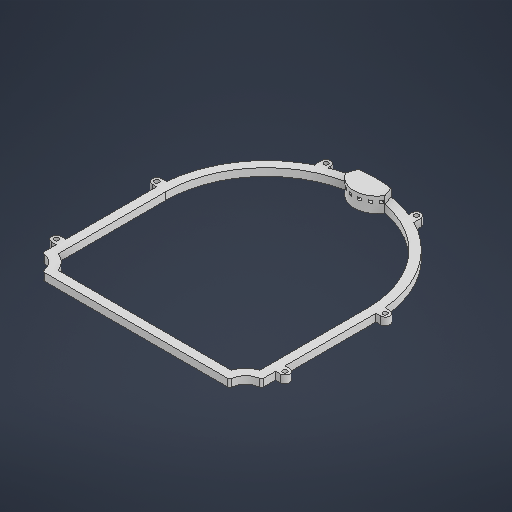
# Autodesk Inventor part: acrylic_clamp
Saved by Autodesk Inventor 2026.2 (Build 302298000, 298)
## iProperties
Created: 2026-04-07
Part Number: acrylic_clamp
Material: Generic
Document SubType Name: Modeling
Designer: Tathagata Sikdar
Density: 1 g/cm^3
Appearance: Default
Author: Tathagata Sikdar
Autodesk Inventor part; units mm, degrees
ref_plane "YZ Plane" through (0, 0, 0) normal (1, 0, 0) x (0, 1, 0)
ref_plane "Work Plane1" through (-76.1962, 17.6834, 72.2477) normal (0, 1, 0) x (-1, 0, 0)
sketch "Sketch1" plane through (-76.1962, 17.6834, 72.2477) normal (0, 1, 0) x (-1, 0, 0)
  arc A0 (-12.9956, -95.0875) -> (-10.7767, -93.6645) centre (-12.6982, -93.1097) ccw projected
  arc A1 (10.7767, -93.6645) -> (-10.7767, -93.6645) centre (0, -96.776) ccw projected
  arc A2 (10.7767, -93.6645) -> (12.9956, -95.0875) centre (12.6982, -93.1097) ccw projected
  arc A3 (12.9956, -95.0875) -> (32.2927, -89.8741) centre (0, -8.6647) ccw projected
  line L0 (32.2927, -89.8741) -> (32.2927, -92.3799) projected
  arc A4 (32.2927, -92.3799) -> (39.7927, -92.3799) centre (36.0427, -92.3799) ccw projected
  line L1 (39.7927, -92.3799) -> (39.7927, -86.4742) projected
  arc A5 (39.7927, -86.4742) -> (87.075, -16.1299) centre (0, -8.6647) ccw projected
  line L2 (87.075, -16.1299) -> (91.0687, -16.1299) projected
  arc A6 (91.0687, -16.1299) -> (91.0687, -8.6299) centre (91.0687, -12.3799) ccw projected
  line L3 (91.0687, -8.6299) -> (87.3944, -8.6299) projected
  line L4 (87.3944, -8.6299) -> (87.3944, 63.8701) projected
  line L5 (87.3944, 63.8701) -> (91.1444, 63.8701) projected
  arc A7 (91.1444, 63.8701) -> (91.1444, 71.3701) centre (91.1444, 67.6201) ccw projected
  line L6 (91.1444, 71.3701) -> (87.3944, 71.3701) projected
  line L7 (87.3944, 71.3701) -> (87.3944, 80.7566) projected
  arc A8 (87.3944, 80.7566) -> (85.666, 82.738) centre (85.3944, 80.7566) ccw projected
  arc A9 (74.7844, 93.6197) -> (85.666, 82.738) centre (87.3944, 95.3481) ccw projected
  arc A10 (74.7844, 93.6197) -> (72.8029, 95.3481) centre (72.8029, 93.3481) ccw projected
  line L8 (72.8029, 95.3481) -> (-72.8029, 95.3481) projected
  arc A11 (-72.8029, 95.3481) -> (-74.7844, 93.6197) centre (-72.8029, 93.3481) ccw projected
  arc A12 (-85.666, 82.738) -> (-74.7844, 93.6197) centre (-87.3944, 95.3481) ccw projected
  arc A13 (-85.666, 82.738) -> (-87.3944, 80.7566) centre (-85.3944, 80.7566) ccw projected
  line L9 (-87.3944, 80.7566) -> (-87.3944, 71.3701) projected
  line L10 (-87.3944, 71.3701) -> (-91.1444, 71.3701) projected
  arc A14 (-91.1444, 71.3701) -> (-91.1444, 63.8701) centre (-91.1444, 67.6201) ccw projected
  line L11 (-91.1444, 63.8701) -> (-87.3944, 63.8701) projected
  line L12 (-87.3944, 63.8701) -> (-87.3944, -8.6299) projected
  line L13 (-87.3944, -8.6299) -> (-91.1444, -8.6299) projected
  arc A15 (-91.1444, -8.6299) -> (-91.1444, -16.1299) centre (-91.1444, -12.3799) ccw projected
  line L14 (-91.1444, -16.1299) -> (-87.075, -16.1299) projected
  arc A16 (-87.075, -16.1299) -> (-39.7927, -86.4742) centre (0, -8.6647) ccw projected
  line L15 (-39.7927, -86.4742) -> (-39.7927, -92.3799) projected
  arc A17 (-39.7927, -92.3799) -> (-32.2927, -92.3799) centre (-36.0427, -92.3799) ccw projected
  line L16 (-32.2927, -92.3799) -> (-32.2927, -89.8741) projected
  arc A18 (-32.2927, -89.8741) -> (-12.9956, -95.0875) centre (0, -8.6647) ccw projected
  circle A19 centre (-36.0427, -92.3799) radius 1.85 projected
  circle A20 centre (91.1444, 67.6201) radius 1.85 projected
  circle A21 centre (36.0427, -92.3799) radius 1.85 projected
  circle A22 centre (-91.1444, 67.6201) radius 1.85 projected
  circle A23 centre (-91.1444, -12.3799) radius 1.85 projected
  circle A24 centre (91.0687, -12.3799) radius 1.85 projected
  arc A25 (85.9744, 79.5665) -> (84.398, 81.5211) centre (83.9744, 79.5665) ccw projected
  line L17 (85.9744, 79.5665) -> (85.9744, -8.6647) projected
  arc A26 (13.9862, -93.4939) -> (85.9744, -8.6647) centre (0, -8.6647) ccw projected
  arc A27 (11.7942, -92.2386) -> (13.9862, -93.4939) centre (13.6608, -91.5205) ccw projected
  arc A28 (11.7942, -92.2386) -> (-11.7942, -92.2386) centre (0, -96.776) ccw projected
  arc A29 (-13.9862, -93.4939) -> (-11.7942, -92.2386) centre (-13.6608, -91.5205) ccw projected
  arc A30 (-85.9744, -8.6647) -> (-13.9862, -93.4939) centre (0, -8.6647) ccw projected
  line L18 (-85.9744, -8.6647) -> (-85.9744, 79.5665) projected
  arc A31 (-84.398, 81.5211) -> (-85.9744, 79.5665) centre (-83.9744, 79.5665) ccw projected
  arc A32 (-84.398, 81.5211) -> (-73.5675, 92.3516) centre (-87.3944, 95.3481) ccw projected
  arc A33 (-71.6128, 93.9281) -> (-73.5675, 92.3516) centre (-71.6128, 91.9281) ccw projected
  line L19 (-71.6128, 93.9281) -> (71.6128, 93.9281) projected
  arc A34 (73.5675, 92.3516) -> (71.6128, 93.9281) centre (71.6128, 91.9281) ccw projected
  arc A35 (73.5675, 92.3516) -> (84.398, 81.5211) centre (87.3944, 95.3481) ccw projected
  arc A36 (14.2722, -87.9193) -> (-14.2722, -87.9193) centre (0, -96.776) ccw projected
  arc A37 (14.2722, -87.9193) -> (16.3718, -88.8243) centre (15.9716, -86.8648) ccw projected
  arc A38 (16.3718, -88.8243) -> (81.8144, -8.6647) centre (0, -8.6647) ccw projected
  line L20 (81.8144, -8.6647) -> (81.8144, 76.5078) projected
  arc A39 (81.8144, 76.5078) -> (80.5609, 78.3633) centre (79.8144, 76.5078) ccw projected
  arc A40 (70.4096, 88.5146) -> (80.5609, 78.3633) centre (87.3944, 95.3481) ccw projected
  arc A41 (70.4096, 88.5146) -> (68.5542, 89.7681) centre (68.5542, 87.7681) ccw projected
  line L21 (68.5542, 89.7681) -> (-68.5542, 89.7681) projected
  arc A42 (-68.5542, 89.7681) -> (-70.4096, 88.5146) centre (-68.5542, 87.7681) ccw projected
  arc A43 (-80.5609, 78.3633) -> (-70.4096, 88.5146) centre (-87.3944, 95.3481) ccw projected
  arc A44 (-80.5609, 78.3633) -> (-81.8144, 76.5078) centre (-79.8144, 76.5078) ccw projected
  line L22 (-81.8144, 76.5078) -> (-81.8144, -8.6647) projected
  arc A45 (-81.8144, -8.6647) -> (-16.3718, -88.8243) centre (0, -8.6647) ccw projected
  arc A46 (-16.3718, -88.8243) -> (-14.2722, -87.9193) centre (-15.9716, -86.8648) ccw projected
  arc A47 (15.6866, -87.5139) -> (80.3944, -8.6647) centre (0, -8.6647) ccw projected
  arc A48 (15.6866, -87.5139) -> (-15.6866, -87.5139) centre (0, -96.776) ccw projected
  arc A49 (-80.3944, -8.6647) -> (-15.6866, -87.5139) centre (0, -8.6647) ccw projected
  line L23 (-80.3944, -8.6647) -> (-80.3944, 76.9038) projected
  arc A50 (-80.3944, 76.9038) -> (-68.9502, 88.3481) centre (-87.3944, 95.3481) ccw projected
  line L24 (-68.9502, 88.3481) -> (68.9502, 88.3481) projected
  arc A51 (68.9502, 88.3481) -> (80.3944, 76.9038) centre (87.3944, 95.3481) ccw projected
  line L25 (80.3944, 76.9038) -> (80.3944, -8.6647) projected
  point P0 (-76.1962, -72.2477)
extrude "Extrusion1" add sketch "Sketch1" along normal blind 6
sketch "Sketch2" plane through (-76.1962, 23.6834, 72.2477) normal (0, 1, 0) x (1, 0, 0)
  line L0 (87.3944, -80.7566) -> (87.3944, -71.3701) projected
  line L1 (87.3944, -71.3701) -> (91.1444, -71.3701) projected
  arc A0 (91.1444, -71.3701) -> (91.1444, -63.8701) centre (91.1444, -67.6201) ccw projected
  line L2 (91.1444, -63.8701) -> (87.3944, -63.8701) projected
  line L3 (87.3944, -63.8701) -> (87.3944, 8.6299) projected
  line L4 (87.3944, 8.6299) -> (91.1444, 8.6299) projected
  arc A1 (91.1444, 8.6299) -> (91.1444, 16.1299) centre (91.1444, 12.3799) ccw projected
  line L5 (91.1444, 16.1299) -> (87.075, 16.1299) projected
  arc A2 (87.075, 16.1299) -> (39.7927, 86.4742) centre (0, 8.6647) ccw projected
  line L6 (39.7927, 86.4742) -> (39.7927, 92.3799) projected
  arc A3 (39.7927, 92.3799) -> (32.2927, 92.3799) centre (36.0427, 92.3799) ccw projected
  line L7 (32.2927, 92.3799) -> (32.2927, 89.8741) projected
  arc A4 (32.2927, 89.8741) -> (12.9956, 95.0875) centre (0, 8.6647) ccw projected
  arc A5 (12.9956, 95.0875) -> (10.7767, 93.6645) centre (12.6982, 93.1097) ccw projected
  arc A6 (-10.7767, 93.6645) -> (10.7767, 93.6645) centre (0, 96.776) ccw projected
  arc A7 (-10.7767, 93.6645) -> (-12.9956, 95.0875) centre (-12.6982, 93.1097) ccw projected
  arc A8 (-12.9956, 95.0875) -> (-32.2927, 89.8741) centre (0, 8.6647) ccw projected
  line L8 (-32.2927, 89.8741) -> (-32.2927, 92.3799) projected
  arc A9 (-32.2927, 92.3799) -> (-39.7927, 92.3799) centre (-36.0427, 92.3799) ccw projected
  line L9 (-39.7927, 92.3799) -> (-39.7927, 86.4742) projected
  arc A10 (-39.7927, 86.4742) -> (-87.075, 16.1299) centre (0, 8.6647) ccw projected
  line L10 (-87.075, 16.1299) -> (-91.0687, 16.1299) projected
  arc A11 (-91.0687, 16.1299) -> (-91.0687, 8.6299) centre (-91.0687, 12.3799) ccw projected
  line L11 (-91.0687, 8.6299) -> (-87.3944, 8.6299) projected
  line L12 (-87.3944, 8.6299) -> (-87.3944, -63.8701) projected
  line L13 (-87.3944, -63.8701) -> (-91.1444, -63.8701) projected
  arc A12 (-91.1444, -63.8701) -> (-91.1444, -71.3701) centre (-91.1444, -67.6201) ccw projected
  line L14 (-91.1444, -71.3701) -> (-87.3944, -71.3701) projected
  line L15 (-87.3944, -71.3701) -> (-87.3944, -80.7566) projected
  arc A13 (-87.3944, -80.7566) -> (-85.666, -82.738) centre (-85.3944, -80.7566) ccw projected
  arc A14 (-74.7844, -93.6197) -> (-85.666, -82.738) centre (-87.3944, -95.3481) ccw projected
  arc A15 (-74.7844, -93.6197) -> (-72.8029, -95.3481) centre (-72.8029, -93.3481) ccw projected
  line L16 (-72.8029, -95.3481) -> (72.8029, -95.3481) projected
  arc A16 (72.8029, -95.3481) -> (74.7844, -93.6197) centre (72.8029, -93.3481) ccw projected
  arc A17 (85.666, -82.738) -> (74.7844, -93.6197) centre (87.3944, -95.3481) ccw projected
  arc A18 (85.666, -82.738) -> (87.3944, -80.7566) centre (85.3944, -80.7566) ccw projected
  arc A19 (-11.7942, 92.2386) -> (11.7942, 92.2386) centre (0, 96.776) ccw projected
  arc A20 (13.9862, 93.4939) -> (11.7942, 92.2386) centre (13.6608, 91.5205) ccw projected
  arc A21 (85.9744, 8.6647) -> (13.9862, 93.4939) centre (0, 8.6647) ccw projected
  line L17 (85.9744, 8.6647) -> (85.9744, -79.5665) projected
  arc A22 (84.398, -81.5211) -> (85.9744, -79.5665) centre (83.9744, -79.5665) ccw projected
  arc A23 (84.398, -81.5211) -> (73.5675, -92.3516) centre (87.3944, -95.3481) ccw projected
  arc A24 (71.6128, -93.9281) -> (73.5675, -92.3516) centre (71.6128, -91.9281) ccw projected
  line L18 (71.6128, -93.9281) -> (-71.6128, -93.9281) projected
  arc A25 (-73.5675, -92.3516) -> (-71.6128, -93.9281) centre (-71.6128, -91.9281) ccw projected
  arc A26 (-73.5675, -92.3516) -> (-84.398, -81.5211) centre (-87.3944, -95.3481) ccw projected
  arc A27 (-85.9744, -79.5665) -> (-84.398, -81.5211) centre (-83.9744, -79.5665) ccw projected
  line L19 (-85.9744, -79.5665) -> (-85.9744, 8.6647) projected
  arc A28 (-13.9862, 93.4939) -> (-85.9744, 8.6647) centre (0, 8.6647) ccw projected
  arc A29 (-11.7942, 92.2386) -> (-13.9862, 93.4939) centre (-13.6608, 91.5205) ccw projected
  circle A30 centre (-91.0687, 12.3799) radius 1.85 projected
  circle A31 centre (91.1444, 12.3799) radius 1.85 projected
  circle A32 centre (91.1444, -67.6201) radius 1.85 projected
  circle A33 centre (-36.0427, 92.3799) radius 1.85 projected
  circle A34 centre (-91.1444, -67.6201) radius 1.85 projected
  circle A35 centre (36.0427, 92.3799) radius 1.85 projected
  line L20 (-81.8144, 8.6647) -> (-81.8144, -76.5078) projected
  arc A36 (-81.8144, -76.5078) -> (-80.5609, -78.3633) centre (-79.8144, -76.5078) ccw projected
  arc A37 (-70.4096, -88.5146) -> (-80.5609, -78.3633) centre (-87.3944, -95.3481) ccw projected
  arc A38 (-70.4096, -88.5146) -> (-68.5542, -89.7681) centre (-68.5542, -87.7681) ccw projected
  line L21 (-68.5542, -89.7681) -> (68.5542, -89.7681) projected
  arc A39 (68.5542, -89.7681) -> (70.4096, -88.5146) centre (68.5542, -87.7681) ccw projected
  arc A40 (80.5609, -78.3633) -> (70.4096, -88.5146) centre (87.3944, -95.3481) ccw projected
  arc A41 (80.5609, -78.3633) -> (81.8144, -76.5078) centre (79.8144, -76.5078) ccw projected
  line L22 (81.8144, -76.5078) -> (81.8144, 8.6647) projected
  arc A42 (81.8144, 8.6647) -> (16.3718, 88.8243) centre (0, 8.6647) ccw projected
  arc A43 (16.3718, 88.8243) -> (14.2722, 87.9193) centre (15.9716, 86.8648) ccw projected
  arc A44 (-14.2722, 87.9193) -> (14.2722, 87.9193) centre (0, 96.776) ccw projected
  arc A45 (-14.2722, 87.9193) -> (-16.3718, 88.8243) centre (-15.9716, 86.8648) ccw projected
  arc A46 (-16.3718, 88.8243) -> (-81.8144, 8.6647) centre (0, 8.6647) ccw projected
  line L23 (80.3944, 8.6647) -> (80.3944, -76.9038) projected
  arc A47 (80.3944, -76.9038) -> (68.9502, -88.3481) centre (87.3944, -95.3481) ccw projected
  line L24 (68.9502, -88.3481) -> (-68.9502, -88.3481) projected
  arc A48 (-68.9502, -88.3481) -> (-80.3944, -76.9038) centre (-87.3944, -95.3481) ccw projected
  line L25 (-80.3944, -76.9038) -> (-80.3944, 8.6647) projected
  arc A49 (-15.6866, 87.5139) -> (-80.3944, 8.6647) centre (0, 8.6647) ccw projected
  arc A50 (-15.6866, 87.5139) -> (15.6866, 87.5139) centre (0, 96.776) ccw projected
  arc A51 (80.3944, 8.6647) -> (15.6866, 87.5139) centre (0, 8.6647) ccw projected
  point P0 (76.1962, 72.2477)
extrude "Extrusion2" add sketch "Sketch2" against normal blind 3.62 contours A18 A17 A16 L16 A15 A14 A13 L15 L14 A12 L13 L12 L11 A11 L10 A10 L9 A9 L8 A8 A7 A6 A5 A4 L7 A3 L6 A2 L5 A1 L4 L3 L2 A0 L1 L0 | A19 A20 A21 L17 A22 A23 A24 L18 A25 A26 A27 L19 A28 A29 | A46 A45 A44 A43 A42 L22 A41 A40 A39 L21 A38 A37 A36 L20
fillet "Fillet1" radius 0.4 28 edges at (-161.7275, 20.0634, 153.0697) (-153.5866, 20.0634, 157.5917) (-149.0646, 20.0634, 165.7325) (-76.1962, 20.0634, 166.1758) (-3.3279, 20.0634, 165.7325) (1.1941, 20.0634, 157.5917) (9.335, 20.0634, 153.0697) (9.7782, 20.0634, 107.6986) (-10.6445, 20.0634, 7.9541) (-63.5293, 20.0634, -21.0084) (-76.1962, 20.0634, -11.8914) (-88.8632, 20.0634, -21.0084) (-141.748, 20.0634, 7.9541) (-162.1707, 20.0634, 107.6986) (-157.6679, 20.0634, 149.8751) (-158.0107, 20.0634, 106.1693) (-139.5723, 20.0634, 11.8425) (-91.3761, 20.0634, -16.4537) (-76.1962, 20.0634, -7.7314) (-61.0163, 20.0634, -16.4537) (-12.8202, 20.0634, 11.8425) (5.6182, 20.0634, 106.1693) (5.2754, 20.0634, 149.8751) (-1.7475, 20.0634, 154.6501) (-6.5225, 20.0634, 161.673) (-76.1962, 20.0634, 162.0158) (-145.87, 20.0634, 161.673) (-150.645, 20.0634, 154.6501)
sketch "Sketch3" plane through (-76.1962, 23.6834, 72.2477) normal (0, 1, 0) x (1, 0, 0)
  arc A0 (80.3944, 8.6647) -> (15.6866, 87.5139) centre (0, 8.6647) ccw projected
  arc A1 (32.2927, 89.8741) -> (12.9956, 95.0875) centre (0, 8.6647) ccw construction
  line L0 (15.6866, 87.5139) -> (12.9956, 95.0875)
  arc A2 (-10.7767, 93.6645) -> (-12.9956, 95.0875) centre (-12.6982, 93.1097) ccw construction
  line L1 (-12.9956, 95.0875) -> (-15.6866, 87.5139)
  arc A3 (-15.6866, 87.5139) -> (15.6866, 87.5139) centre (0, 96.776) ccw
  arc A4 (-15.6866, 87.5139) -> (15.6866, 87.5139) centre (0, 96.776) ccw construction
  arc A5 (12.9956, 95.0875) -> (10.7767, 93.6645) centre (12.6982, 93.1097) ccw construction
  arc A6 (12.9956, 95.0875) -> (-12.9956, 95.0875) centre (0, 8.6647) ccw
  arc A7 (-12.9956, 95.0875) -> (-32.2927, 89.8741) centre (0, 8.6647) ccw projected
  point P0 (76.1962, 72.2477)
  constraints: 4 end point, 4 point on circle, 2 centre point, 2 concentric, 1 coincident
extrude "Extrusion3" add sketch "Sketch3" along normal blind 12 from surface at -6
ref_plane "Work Plane2" through (-76.1962, 26.6834, -24.5283) normal (0, 1, 0) x (1, 0, 0)
sketch "Sketch4" plane through (-76.1962, 26.6834, -24.5283) normal (0, 1, 0) x (1, 0, 0)
  arc A0 (-15.6866, -9.2621) -> (15.6866, -9.2621) centre (0, 0) ccw projected
  arc A1 (-6, -4.3224) -> (6, -4.3224) centre (0, -0.7169) ccw
  arc A2 (32.2927, -6.9019) -> (-32.2927, -6.9019) centre (0, -88.1113) ccw construction
  line L0 (6, -4.3224) -> (-6, -4.3224)
  line L1 (-6, -4.3224) -> (-15.2891, -9.9045)
  line L2 (-5.4398, -5.1224) -> (-13.7994, -11.8925)
  line L3 (-3.3398, -6.8688) -> (-8.4723, -16.3226)
  line L4 (-4.1635, -6.3441) -> (-10.6093, -15.056)
  line L5 (-0.7314, -7.6786) -> (-1.8553, -18.3769)
  line L6 (-1.6931, -7.509) -> (-4.3144, -18.0245)
  line L7 (1.9884, -7.4285) -> (5.0441, -17.7426)
  line L8 (1.035, -7.64) -> (2.6374, -18.3581)
  line L9 (4.4055, -6.1567) -> (11.1756, -14.5163)
  line L10 (3.6056, -6.7169) -> (9.1876, -16.006)
  line L11 (6, -4.3224) -> (15.2891, -9.9045)
  line L12 (5.4398, -5.1224) -> (13.7994, -11.8925)
  point P0 (76.1962, -24.5283)
  point P1 (0, -7.7169)
  point P2 (-4.1635, -6.3441)
  point P3 (-10.4894, -14.8939)
  point P4 (-8.3895, -16.1701)
  point P5 (-3.3398, -6.8688)
  point P6 (-1.6931, -7.509)
  point P7 (-4.2378, -17.7171)
  point P8 (-1.8288, -18.1249)
  point P9 (-0.7314, -7.6786)
  point P10 (1.035, -7.64)
  point P11 (2.5886, -18.032)
  point P12 (4.9791, -17.5232)
  point P13 (1.9884, -7.4285)
  point P14 (3.6056, -6.7169)
  point P15 (9.0647, -15.8015)
  point P16 (11.1108, -14.4363)
  point P17 (4.4055, -6.1567)
  dimension "d8" = 7
  dimension "d9" = 6
  dimension "d14" = 8
  dimension "d17" = 90
  dimension "d19" = 8
  constraints: 26 end point, 10 point on circle, 4 line through centre, 1 centre point, 1 horizontal, 1 vertical alignment, 25 other
  measures "d8" radius of A1
  measures "d9" horizontal distance of L0.start point (0, -7.717)
  measures "d14" angle of L2 L1
  measures "d19" angle of L11 L12
extrude "Extrusion4" cut sketch "Sketch4" against normal blind 2 contours L1 A1 L2 A0 | L0 A1 | L4 A1 L3 A0 | L11 A0 L12 A1 | L6 A1 L5 A0 | L9 A0 L10 A1 | L8 A1 L7 A0
sketch "Sketch5" plane through (-82.1962, 26.6834, -20.2059) normal (0, 0, 1) x (1, 0, 0)
  line L0 (5.2686, -2) -> (7.035, -2) projected
  circle A0 centre (6.1518, -2) radius 3.9
  point P0 (82.1962, -26.6834)
  dimension "d22" = 7.8
  constraints: 1 centre point, 1 midpoint
  measures "d22" diameter of A0
extrude "Extrusion5" cut sketch "Sketch5" against normal through all
body "Solid1"
